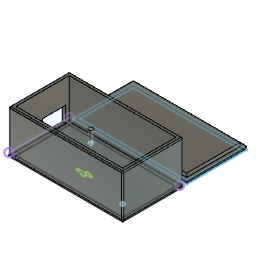
esp32 thund last v1 (Autodesk Fusion 360 design; units mm, degrees)
Autodesk Fusion 360 part; units mm, degrees
sketch "Sketch1" plane through (0, 0, 0) normal (0, 0, 1) x (1, 0, 0)
  line L0 (0, 0) -> (60, 0)
  line L1 (60, 0) -> (60, 30)
  line L2 (60, 30) -> (0, 30)
  line L3 (0, 30) -> (0, 0)
  line L4 (-2, -2) -> (62, -2)
  line L5 (62, -2) -> (62, 32)
  line L6 (62, 32) -> (-2, 32)
  line L7 (-2, 32) -> (-2, -2)
  dimension "d1" = 60
  dimension "d2" = 30
  dimension "d3" = 2
  constraint horizontal L0
  constraint vertical L1
  constraint horizontal L2
  constraint vertical L3
  constraint coincident L0.start L3.end
  measures "d1" distance of L0.start L0.end
  measures "d2" distance of L0.start L2.end
extrude "Extrude1" add sketch "Sketch1" along normal blind 1.5 contours L0 L1 L2 L3 makes body 1
extrude "Extrude2" add sketch "Sketch1" along normal blind 24 bodies 1
sketch "Sketch2" plane through (62, 0, 0) normal (1, 0, 0) x (0, 1, 0)
  line L0 (-2, 0) -> (32, 0)
  line L1 (32, 0) -> (32, 24)
  line L2 (32, 24) -> (-2, 24)
  line L3 (-2, 24) -> (-2, 0)
  point P0 (30, 1.5)
sketch "Sketch3" plane through (-2, 0, 0) normal (-1, 0, 0) x (0, -1, 0)
  line L0 (-32, 0) -> (2, 0)
  line L1 (2, 0) -> (2, 24)
  line L2 (2, 24) -> (-32, 24)
  line L3 (-32, 24) -> (-32, 0)
sketch "Sketch1 (2)" plane through (0, 0, 0) normal (0, 0, 1) x (1, 0, 0) in component "cover"
  line L0 (-2, 34) -> (62, 34)
  line L1 (62, 34) -> (62, 68)
  line L2 (62, 68) -> (-2, 68)
  line L3 (-2, 68) -> (-2, 34)
  line L4 (0, 36) -> (60, 36)
  line L5 (60, 36) -> (60, 66)
  line L6 (60, 66) -> (0, 66)
  line L7 (0, 66) -> (0, 36)
  dimension "d21" = 64
  dimension "d22" = 34
  dimension "d23" = -2
  constraint horizontal L0
  constraint vertical L1
  constraint horizontal L2
  constraint vertical L3
  measures "d21" distance of L0.start L0.end
  measures "d22" distance of L0.start L2.end
extrude "Extrude1'" add sketch "Sketch1 (2)" along normal blind 3.5 separate body contours L4 L5 L6 L7 makes body 2 in component "cover"
extrude "Extrude2'" add sketch "Sketch1 (2)" along normal blind 1.5 bodies 2 in component "cover"
sketch "Sketch4" plane through (0, 0, 0) normal (0, 0, 1) x (1, 0, 0)
  line L0 (-2, 34) -> (62, 34)
  line L1 (62, 34) -> (62, 68)
sketch "Sketch5" plane through (0, 0, 0) normal (0, 0, 1) x (1, 0, 0)
sketch "Sketch7" plane through (0, 0, 1.5) normal (0, 0, 1) x (-1, 0, 0)
  line L0 (0, -30) -> (0, 0)
  line L1 (0, 0) -> (-60, 0)
  line L2 (-60, 0) -> (-60, -30)
  line L3 (-60, -30) -> (0, -30)
  circle A0 centre (-55, -5) radius 1.25
  circle A1 centre (-16.5, -25.7) radius 1.25
  line L4 (2, -32) -> (2, 2)
  spline S0 degree 3 poles (-24.9969, -9.3105) (-24.9532, -9.2408) (-24.9445, -9.1603) (-24.9726, -9.0832) knots 0 0 0 0 1 1 1 1
  spline S1 degree 3 poles (-24.9726, -9.0832) (-25.0142, -8.969) (-25.1468, -8.7941) (-25.8151, -8.596) knots 0 0 0 0 1 1 1 1
  line L5 (-25.8151, -8.596) -> (-29.1072, -7.6203)
  spline S2 degree 3 poles (-29.1072, -7.6203) (-29.9325, -7.3756) (-30.5651, -7.3786) (-30.7999, -7.6281) knots 0 0 0 0 1 1 1 1
  spline S3 degree 3 poles (-30.7999, -7.6281) (-30.9023, -7.7369) (-30.9267, -7.8847) (-30.8687, -8.0441) knots 0 0 0 0 1 1 1 1
  line L6 (-30.8687, -8.0441) -> (-30.6404, -8.6715)
  line L7 (-30.6404, -8.6715) -> (-32.3981, -8.94)
  spline S4 degree 3 poles (-32.3981, -8.94) (-32.8976, -9.0165) (-33.1913, -9.1394) (-33.2959, -9.3156) knots 0 0 0 0 1 1 1 1
  spline S5 degree 3 poles (-33.2959, -9.3156) (-33.3423, -9.3939) (-33.3509, -9.4839) (-33.3201, -9.5687) knots 0 0 0 0 1 1 1 1
  spline S6 degree 3 poles (-33.3201, -9.5687) (-33.249, -9.7638) (-32.974, -9.9314) (-32.479, -10.0813) knots 0 0 0 0 1 1 1 1
  line L8 (-32.479, -10.0813) -> (-31.0194, -10.5228)
  spline S7 degree 3 poles (-31.0194, -10.5228) (-30.674, -10.6273) (-29.524, -10.9436) (-29.2271, -10.6298) knots 0 0 0 0 1 1 1 1
  spline S8 degree 3 poles (-29.2271, -10.6298) (-29.1554, -10.554) (-29.1364, -10.4495) (-29.175, -10.3435) knots 0 0 0 0 1 1 1 1
  line L9 (-29.175, -10.3435) -> (-29.3148, -9.9595)
  line L10 (-29.3148, -9.9595) -> (-25.9131, -9.6243)
  spline S9 degree 3 poles (-25.9131, -9.6243) (-25.2264, -9.5566) (-25.0614, -9.4128) (-24.9969, -9.3105) knots 0 0 0 0 1 1 1 1
  line L11 (-25.9412, -9.3379) -> (-29.5274, -9.6912)
  spline S10 degree 3 poles (-29.5274, -9.6912) (-29.5716, -9.6957) (-29.6114, -9.7201) (-29.635, -9.7578) knots 0 0 0 0 1 1 1 1
  spline S11 degree 3 poles (-29.635, -9.7578) (-29.6587, -9.7955) (-29.6637, -9.8419) (-29.6485, -9.8837) knots 0 0 0 0 1 1 1 1
  line L12 (-29.6485, -9.8837) -> (-29.4467, -10.4403)
  spline S12 degree 3 poles (-29.4467, -10.4403) (-29.5487, -10.5053) (-30.0567, -10.513) (-30.936, -10.2471) knots 0 0 0 0 1 1 1 1
  line L13 (-30.936, -10.2471) -> (-32.3955, -9.8056)
  spline S13 degree 3 poles (-32.3955, -9.8056) (-32.8674, -9.6629) (-33.0287, -9.5277) (-33.0508, -9.4675) knots 0 0 0 0 1 1 1 1
  spline S14 degree 3 poles (-33.0508, -9.4675) (-33.0504, -9.4659) (-32.9899, -9.3216) (-32.3548, -9.2244) knots 0 0 0 0 1 1 1 1
  line L14 (-32.3548, -9.2244) -> (-30.4236, -8.9293)
  spline S15 degree 3 poles (-30.4236, -8.9293) (-30.3809, -8.9228) (-30.3435, -8.8974) (-30.3215, -8.8605) knots 0 0 0 0 1 1 1 1
  spline S16 degree 3 poles (-30.3215, -8.8605) (-30.2997, -8.8234) (-30.2954, -8.7783) (-30.3101, -8.7379) knots 0 0 0 0 1 1 1 1
  line L15 (-30.3101, -8.7379) -> (-30.5984, -7.9457)
  spline S17 degree 3 poles (-30.5984, -7.9457) (-30.6278, -7.865) (-30.6026, -7.8384) (-30.5905, -7.8254) knots 0 0 0 0 1 1 1 1
  spline S18 degree 3 poles (-30.5905, -7.8254) (-30.4887, -7.7171) (-30.0313, -7.6465) (-29.1891, -7.8962) knots 0 0 0 0 1 1 1 1
  line L16 (-29.1891, -7.8962) -> (-25.8967, -8.8719)
  spline S19 degree 3 poles (-25.8967, -8.8719) (-25.4095, -9.0163) (-25.2824, -9.1307) (-25.2519, -9.1685) knots 0 0 0 0 1 1 1 1
  spline S20 degree 3 poles (-25.2519, -9.1685) (-25.289, -9.1998) (-25.4356, -9.288) (-25.9412, -9.3379) knots 0 0 0 0 1 1 1 1
  dimension "d35" = 2.5
  dimension "d36" = 2.5
  dimension "d52" = 18.5
  measures "d35" diameter of A0
  measures "d36" diameter of A1
  measures "d52" distance of A1.centre L4
extrude "Extrude12" cut sketch "Sketch7" against normal blind 2.5 contours L11 S10 S11 L12 S12 L13 S13 S14 L14 S15 S16 L15 S17 S18 L16 S19 S20 bodies 1
extrude "Extrude6" add sketch "Sketch7" along normal blind 7 contours A1 bodies 1
extrude "Extrude7" add sketch "Sketch7" along normal blind 7 contours A0 bodies 1
sketch "Sketch8" plane through (-2, 15, 12) normal (-1, 0, 0) x (0, -1, 0)
  line L0 (-13, -10.4362) -> (0, -10.4362)
  line L1 (0, -10.4362) -> (0, -1.4362)
  line L2 (0, -1.4362) -> (-13, -1.4362)
  line L3 (-13, -1.4362) -> (-13, -10.4362)
  point P0 (-17, -10.5)
  dimension "d47" = 13
  dimension "d48" = 9
  dimension "d57" = 4
  constraint horizontal L0
  constraint vertical L1
  constraint horizontal L2
  constraint vertical L3
  measures "d47" distance of L0.start L0.end
  measures "d48" distance of L0.start L2.end
  measures "d57" horizontal distance of L0.start P0
extrude "Extrude10" cut sketch "Sketch8" against normal blind 2.5 bodies 1
fillet "Fillet1" radius 0.6 1 edges at (-2, 15, 24) on bodies 1
fillet "Fillet2" radius 0.6 3 edges at (-2, -2, 11.7) (-1.8243, -2, 23.8243) (30.3, -2, 24) on bodies 1
fillet "Fillet3" radius 0.6 3 edges at (-2, 15.3, 0) (-1.8243, -1.8243, 0) (30.3, -2, 0) on bodies 1
fillet "Fillet4" radius 0.6 5 edges at (30.3, 32, 0) (-1.8243, 32, 0.1757) (-2, 32, 12) (-1.8243, 32, 23.8243) (30.3, 32, 24) on bodies 1
fillet "Fillet5" radius 0.6 8 edges at (62, 31.8243, 23.8243) (62, 15, 24) (62, -1.8243, 23.8243) (62, -2, 12) (62, -1.8243, 0.1757) (62, 15, 0) (62, 31.8243, 0.1757) (62, 32, 12) on bodies 1
fillet "Fillet1'" radius 0.6 1 edges at (62, 51, 0) on bodies 2 in component "cover"
fillet "Fillet2'" radius 0.6 3 edges at (29.7, 34, 0) (61.8243, 34, 0.1757) (62, 34, 1.05) on bodies 2 in component "cover"
fillet "Fillet3'" radius 0.6 3 edges at (-2, 51.3, 0) (-2, 34.1757, 0.1757) (-2, 34, 1.05) on bodies 2 in component "cover"
fillet "Fillet4'" radius 0.6 5 edges at (62, 68, 1.05) (61.8243, 68, 0.1757) (30, 68, 0) (-1.8243, 68, 0.1757) (-2, 68, 1.05) on bodies 2 in component "cover"
sketch "Sketch9" plane through (0, 0, 1.5) normal (0, 0, 1) x (-1, 0, 0)
component "cover" placed x (1, 0, 0) y (0, 1, 0) z (0, 0, 1) at (0, 0, 0)
